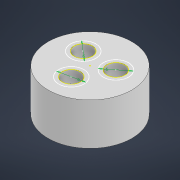
# Autodesk Inventor part: Fahrwerk_Fix_test
Saved by Autodesk Inventor 2021 (Build 250183000, 183)
## iProperties
Created: 2021-03-06
Part Number: Fahrwerk_Fix_test
Material: Generisch
Document SubType Name: Modeling
Designer: Ctroi
Density: 1 g/cm^3
Appearance: Vorgabe
Author: Ctroi
Autodesk Inventor part; units mm, degrees
ref_plane "YZ Plane" through (0, 0, 0) normal (1, 0, 0) x (0, 1, 0)
ref_plane "XZ Plane" through (0, 0, 0) normal (0, 1, 0) x (-1, 0, 0)
ref_plane "XY Plane" through (0, 0, 0) normal (0, 0, 1) x (1, 0, 0)
sketch "Skizze1" plane through (0, 0, 0) normal (0, 1, 0) x (-1, 0, 0)
  circle A0 centre (0, 0) radius 10
  dimension "d0" = 20
  constraints: 1 centre point, 1 coincident
  measures "d0" diameter of A0
extrude "Extrusion1" add sketch "Skizze1" along normal blind 10
sketch "Skizze2" plane through (0, 10, 0) normal (0, 1, 0) x (1, 0, 0)
  line L0 (14, 0) -> (-14, 0) projected
  line L1 (0, 14) -> (0, -14) projected
  line L2 (-3.8971, 2.25) -> (0, 0)
  line L3 (0, 0) -> (3.8971, 2.25)
  line L4 (0, 0) -> (0, -4.5)
  circle A0 centre (-3.8971, 2.25) radius 2.15
  circle A1 centre (3.8971, 2.25) radius 2.15
  circle A2 centre (0, -4.5) radius 2.15
  dimension "d17" = 4.5
  dimension "d18" = 4.5
  dimension "d19" = 4.5
  dimension "d20" = 120
  dimension "d21" = 120
  dimension "d22" = 4.3
  dimension "d23" = 4.3
  dimension "d24" = 4.3
  constraints: 6 end point, 3 centre point, 3 coincident, 1 point on line
  measures "d17" distance of L2.end L4.end
  measures "d18" distance of L2.end L3.end
  measures "d19" distance of L2.end L2.start
  measures "d20" angle of L1 L2
  measures "d21" angle of L1 L3
  measures "d22" diameter of A0
  measures "d23" diameter of A1
  measures "d24" diameter of A2
extrude "Extrusion3" cut sketch "Skizze2" against normal blind 6
sketch "Skizze3" plane through (0, 10, 0) normal (0, 1, 0) x (1, 0, 0)
  circle A0 centre (-3.8971, 2.25) radius 2.15 projected
  circle A1 centre (3.8971, 2.25) radius 2.15 projected
  circle A2 centre (0, -4.5) radius 2.15 projected
  circle A3 centre (-3.8971, 2.25) radius 2.15 projected
  circle A4 centre (-3.8971, 2.25) radius 3
  circle A5 centre (3.8971, 2.25) radius 3
  circle A6 centre (0, -4.5) radius 3
  point P0 (0, 0)
  dimension "d27" = 6
  dimension "d28" = 6
  dimension "d29" = 6
  constraints: 3 centre point, 3 coincident
  measures "d27" diameter of A4
  measures "d28" diameter of A5
  measures "d29" diameter of A6
